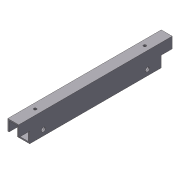
# Autodesk Inventor part: Frame_MainHorizontalMount
Saved by Autodesk Inventor 2012 (Build 160160000, 160)
## iProperties
Created: 2012-01-14
Part Number: Frame_MainHorizontalMount
Material: Aluminum-6061
Document SubType Name: Modeling
Designer: JesseK
Mass: 393.908 g
Surface Area: 932.775 cm^2
Volume: 145.353 cm^3
Density: 2.71 g/cm^3
Author: JesseK
Autodesk Inventor part; units mm, degrees
ref_plane "YZ Plane" through (0, 0, 0) normal (1, 0, 0) x (0, 1, 0)
ref_plane "XZ Plane" through (0, 0, 0) normal (0, 1, 0) x (-1, 0, 0)
ref_plane "XY Plane" through (0, 0, 0) normal (0, 0, 1) x (1, 0, 0)
sketch "Sketch1" plane through (0, 0, 0) normal (0, 0, 1) x (1, 0, 0)
  line L0 (0, 0) -> (25.4, 0)
  line L1 (25.4, 0) -> (25.4, 50.8)
  line L2 (25.4, 50.8) -> (0, 50.8)
  line L3 (0, 50.8) -> (0, 0)
  dimension "d0" = 25.4
  dimension "d1" = 50.8
  constraints: 8 end point, 2 parallel, 1 horizontal, 1 perpendicular
  measures "d0" distance of L1.end L2.end
  measures "d1" distance of L2.end L0.start
extrude "Extrusion1" add sketch "Sketch1" along normal blind 355.6
shell "Shell1" thickness 3.175 removed faces 2 at (16.9333, 16.9333, 0) at (8.4667, 33.8667, 355.6)
sketch "Sketch2" plane through (25.4, 0, 0) normal (1, 0, 0) x (0, 0, -1)
  line L0 (-355.6, 0) -> (-330.2, 0)
  line L1 (-330.2, 0) -> (-330.2, 25.4)
  line L2 (-330.2, 25.4) -> (-355.6, 25.4)
  line L3 (-355.6, 25.4) -> (-355.6, 0)
  line L4 (0, 0) -> (-25.4, 0)
  line L5 (-25.4, 0) -> (-25.4, 25.4)
  line L6 (-25.4, 25.4) -> (0, 25.4)
  line L7 (0, 25.4) -> (0, 0)
  dimension "d5" = 25.4
  constraints: 16 end point, 4 parallel, 2 equal length, 2 horizontal, 2 perpendicular, 1 collinear
  measures "d5" distance of L1.end L2.end
extrude "Extrusion2" cut sketch "Sketch2" against normal through all
sketch "Sketch3" plane through (25.4, 50.8, 355.6) normal (1, 0, 0) x (0, 0, -1)
  line L0 (330.2, -50.8) -> (330.2, -25.4) projected
  line L1 (25.4, -25.4) -> (25.4, -50.8) projected
  line L2 (330.2, -50.8) -> (25.4, -50.8) projected
  circle A0 centre (57.15, -38.1) radius 4.7625
  circle A1 centre (298.45, -38.1) radius 4.7625
  point P0 (355.6, -50.8)
  dimension "d8" = 9.525
  dimension "d9" = 31.75
  dimension "d10" = 12.7
  dimension "d11" = 12.7
  dimension "d12" = 31.75
  constraints: 2 centre point, 1 equal radius
  measures "d8" diameter of A0
  measures "d9" distance from line of L1 A0.centre
  measures "d10" distance from line of L2 A0.centre
  measures "d11" distance from line of L2 A1.centre
  measures "d12" distance from line of L0 A1.centre
extrude "Extrusion3" cut sketch "Sketch3" against normal through all
sketch "Sketch4" plane through (0, 50.8, 0) normal (0, 1, 0) x (1, 0, 0)
  line L0 (0, -355.6) -> (25.4, -355.6)
  line L1 (25.4, 0) -> (0, 0) projected
  line L2 (0, 0) -> (0, -355.6) projected
  circle A0 centre (12.7, -50.8) radius 3.175
  circle A1 centre (12.7, -304.8) radius 3.175
  line L3 (12.7, 0) -> (12.7, -50.8) construction
  line L4 (12.7, -50.8) -> (12.7, -304.8) construction
  line L5 (12.7, -304.8) -> (12.7, -355.6) construction
  dimension "d15" = 6.35
  dimension "d16" = 12.7
  dimension "d17" = 50.8
  dimension "d18" = 254
  dimension "d19" = 50.8
  constraints: 8 end point, 2 centre point, 2 midpoint, 1 equal radius, 1 vertical
  measures "d15" diameter of A0
  measures "d16" distance from line of L2 L3.end
  measures "d17" distance of L3.start L3.end
  measures "d18" distance of L3.end L4.end
  measures "d19" distance of L4.end L5.end
extrude "Extrusion4" cut sketch "Sketch4" against normal up to next
body "Solid1"
